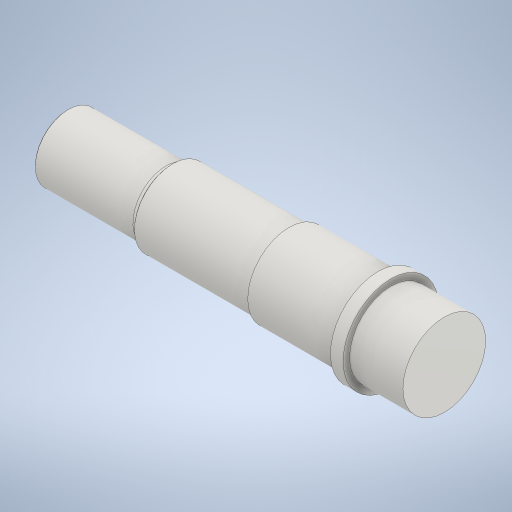
# Autodesk Inventor part: ТихВал
Saved by Autodesk Inventor 2023.2 (Build 272271000, 271)
## iProperties
CustomPartVersion: 1
Created: 2023-10-14
Part Number: ТихВал
Material: Steel
Document SubType Name: Modeling
Designer: Vovan
Density: 1 g/cm^3
Appearance: Steel
Length: 296,000 мм
Author: Vovan
Autodesk Inventor part; units mm, degrees
ref_plane "Начальная плоскость" through (0, 0, 0) normal (1, 0, 0) x (0, 1, 0)
ref_plane "XZ Plane" through (0, 0, 0) normal (0, 1, 0) x (-1, 0, 0)
ref_plane "XY Plane" through (0, 0, 0) normal (0, 0, 1) x (1, 0, 0)
sketch "Основной эскиз" plane through (0, 0, 0) normal (0, 0, 1) x (1, 0, 0)
  line L0 (0, 0) -> (296, 0)
  line L1 (0, 0) -> (0, 26)
  line L2 (0, 26) -> (82, 26)
  line L3 (82, 26) -> (82, 30)
  line L4 (82, 30) -> (174, 30)
  line L5 (174, 30) -> (174, 32.5)
  line L6 (174, 32.5) -> (244, 32.5)
  line L7 (244, 32.5) -> (244, 37.5)
  line L8 (254, 37.5) -> (254, 32.5)
  line L9 (244, 37.5) -> (254, 37.5)
  line L10 (296, 32.5) -> (296, 0)
  line L11 (254, 32.5) -> (296, 32.5)
  dimension "d3" = 52
  dimension "d4" = 60
  dimension "d5" = 65
  dimension "d6" = 75
  dimension "d7" = 65
  constraints: 24 end point, 7 horizontal, 6 vertical
  measures "d3" diameter of L2 L0
  measures "d4" diameter of L4 L0
  measures "d5" diameter of L6 L0
  measures "d6" diameter of L9 L0
  measures "d7" diameter of L11 L0
revolve "Вращение1" add sketch "Основной эскиз" angle 360 about axis through (0, 0, 0) along (1, 0, 0)
chamfer "Фаска3" distance 0.5 angle 45 1 edges at (82, -30, 0) measured on face at (143.3333, 29.9027, -2.414)
chamfer "Фаска1" distance 0.5 angle 45 1 edges at (0, -26, 0) measured on face at (54.6667, 25.9157, -2.0921)
fillet "Сопряжение1" radius 5 1 edges at (82, -26, 0)
equation "\"Length\" = 296"
